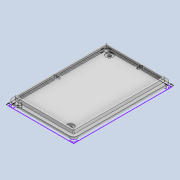
# Autodesk Inventor part: proper shit spodnji
Saved by Autodesk Inventor 2020 (Build 240168000, 168)
## iProperties
Created: 2020-08-03
Part Number: proper shit spodnji
Material: Generic
Document SubType Name: Modeling
Designer: borbu
Density: 1 g/cm^3
Appearance: Default
Author: borbu
Autodesk Inventor part; units mm, degrees
ref_plane "YZ Plane" through (0, 0, 0) normal (1, 0, 0) x (0, 1, 0)
ref_plane "XZ Plane" through (0, 0, 0) normal (0, 1, 0) x (-1, 0, 0)
ref_plane "XY Plane" through (0, 0, 0) normal (0, 0, 1) x (1, 0, 0)
sketch "Sketch1" plane through (0, 0, 0) normal (0, 1, 0) x (-1, 0, 0)
  line L0 (-25, 37.5) -> (25, 37.5)
  line L1 (25, 37.5) -> (25, -37.5)
  line L2 (25, -37.5) -> (-25, -37.5)
  line L3 (-25, -37.5) -> (-25, 37.5)
  line L4 (25, 37.5) -> (-25, -37.5) construction
  line L5 (-22.5, 35) -> (22.5, 35)
  line L6 (22.5, 35) -> (22.5, -35)
  line L7 (22.5, -35) -> (-22.5, -35)
  line L8 (-22.5, -35) -> (-22.5, 35)
  line L9 (22.5, 35) -> (-22.5, -35) construction
  line L10 (22.5, 35) -> (20, 35)
  line L11 (20, 35) -> (20, 32.5)
  line L12 (20, 32.5) -> (22.5, 32.5)
  line L13 (22.5, 32.5) -> (22.5, 35)
  arc A0 (22.5, 32.5) -> (20, 35) centre (20, 32.5) ccw
  line L14 (25, 37.5) -> (21.5, 37.5)
  line L15 (21.5, 37.5) -> (21.5, 34)
  line L16 (21.5, 34) -> (25, 34)
  line L17 (25, 34) -> (25, 37.5)
  line L18 (22.5, -35) -> (20, -35)
  line L19 (20, -35) -> (20, -32.5)
  line L20 (20, -32.5) -> (22.5, -32.5)
  line L21 (22.5, -32.5) -> (22.5, -35)
  line L22 (-22.5, -35) -> (-20, -35)
  line L23 (-20, -35) -> (-20, -32.5)
  line L24 (-20, -32.5) -> (-22.5, -32.5)
  line L25 (-22.5, -32.5) -> (-22.5, -35)
  line L26 (-22.5, 35) -> (-20, 35)
  line L27 (-20, 35) -> (-20, 32.5)
  line L28 (-20, 32.5) -> (-22.5, 32.5)
  line L29 (-22.5, 32.5) -> (-22.5, 35)
  arc A1 (-20, 35) -> (-22.5, 32.5) centre (-20, 32.5) ccw
  arc A2 (-22.5, -32.5) -> (-20, -35) centre (-20, -32.5) ccw
  arc A3 (20, -35) -> (22.5, -32.5) centre (20, -32.5) ccw
  arc A4 (25, 34) -> (21.5, 37.5) centre (21.5, 34) ccw
  line L30 (25, -37.5) -> (21.5, -37.5)
  line L31 (21.5, -37.5) -> (21.5, -34)
  line L32 (21.5, -34) -> (25, -34)
  line L33 (25, -34) -> (25, -37.5)
  line L34 (-25, -37.5) -> (-21.5, -37.5)
  line L35 (-21.5, -37.5) -> (-21.5, -34)
  line L36 (-21.5, -34) -> (-25, -34)
  line L37 (-25, -34) -> (-25, -37.5)
  line L38 (-25, 37.5) -> (-21.5, 37.5)
  line L39 (-21.5, 37.5) -> (-21.5, 34)
  line L40 (-21.5, 34) -> (-25, 34)
  line L41 (-25, 34) -> (-25, 37.5)
  arc A5 (-21.5, 37.5) -> (-25, 34) centre (-21.5, 34) ccw
  arc A6 (-25, -34) -> (-21.5, -37.5) centre (-21.5, -34) ccw
  arc A7 (21.5, -37.5) -> (25, -34) centre (21.5, -34) ccw
  point P0 (0, 0)
  point P1 (25, 34)
  point P2 (-25, -34)
  point P3 (-22.5, -32.5)
  point P4 (-22, -34)
  point P5 (-22.5, -34)
  point P6 (22.5, -32.5)
  dimension "d0" = 50
  dimension "d1" = 75
  dimension "d2" = 45
  dimension "d3" = 70
  dimension "d8" = 2.5
  dimension "d9" = 2.5
  constraints: 84 end point, 20 parallel, 16 point on circle, 10 horizontal, 10 perpendicular, 8 centre point, 8 coincident, 2 midpoint, 1 point on line
  measures "d0" distance of L1.end L2.end
  measures "d1" distance of L0.end L1.end
  measures "d2" distance of L6.end L7.end
  measures "d3" distance of L5.end L6.end
  measures "d8" distance of L12.end L11.end
  measures "d9" distance of L11.end L10.end
extrude "Extrusion3" add sketch "Sketch1" along normal blind 3.5 contours L0 L15 L5 L39 | L39 L5 L8 L40 A5 | L40 L8 L36 L3 | A4 L16 L6 L5 L15 | L39 A1 L40 L8 L5 | L5 A1 L39 | L36 L8 L7 L35 A6 | L40 A1 L8 | L15 A0 L5 | L5 L6 L16 A0 L15 | L1 L32 L6 L16 | L5 L11 L12 L6 L20 L19 L7 L23 L24 L8 L28 L27 | L27 L28 A1 L40 L39 | L39 L40 A1 | L36 A2 L35 L7 L8 | L8 A2 L36 | L35 L7 L31 L2 | A0 L15 L16 L12 L11 | A0 L16 L15 | A7 L31 L7 L6 L32 | L6 A0 L16 | L24 L23 A2 L35 L36 | L36 L35 A2 | L35 A2 L7 | L32 A3 L6 | L6 L7 L31 A3 L32 | L7 A3 L31 | A3 L32 L31 L19 L20 | A3 L31 L32
fillet "Fillet1" radius 3 8 edges at (-23.9749, 0, 36.4749) (0, 0, 37.5) (23.9749, 0, 36.4749) (25, 0, 0) (23.9749, 0, -36.4749) (0, 0, -37.5) (-23.9749, 0, -36.4749) (-25, 0, 0)
sketch "Sketch2" plane through (0, 3.5, 0) normal (0, 1, 0) x (1, 0, 0)
  arc A0 (20, 32.5) -> (17.5, 35) centre (17.5, 32.5) ccw projected
  line L0 (17.5, 35) -> (17.5, 33.5)
  line L1 (20, -32.5) -> (20, 32.5) projected
  line L2 (20, 32.5) -> (18.5, 32.5)
  line L3 (18.5, 32.5) -> (17.5, 33.5)
  line L4 (18, 33) -> (16.0555, 31.0555)
  circle A1 centre (16.0555, 31.0555) radius 2.75
  line L5 (-20, 32.5) -> (-20, -32.5) projected
  line L6 (-20, -32.5) -> (-18.5, -32.5)
  line L7 (-17.5, -35) -> (17.5, -35) projected
  line L8 (-17.5, -35) -> (-17.5, -33.5)
  line L9 (-17.5, -33.5) -> (-18.5, -32.5)
  line L10 (-18, -33) -> (-16.0555, -31.0555)
  line L11 (-18, -33) -> (-15.25, -33) construction
  circle A2 centre (-16.0555, -31.0555) radius 2.75
  arc A3 (17.5812, 28.7675) -> (18.8055, 31.0555) centre (16.0555, 31.0555) ccw construction
  arc A4 (17.8504, 28.3639) -> (19.2906, 31.0555) centre (16.0555, 31.0555) ccw
  arc A5 (17.3121, 29.1712) -> (18.3203, 31.0555) centre (16.0555, 31.0555) ccw
  arc A6 (17.3121, 29.1712) -> (17.8504, 28.3639) centre (17.5812, 28.7675) ccw
  arc A7 (19.2906, 31.0555) -> (18.3203, 31.0555) centre (18.8055, 31.0555) ccw
  arc A8 (14.2605, 33.747) -> (12.8203, 31.0555) centre (16.0555, 31.0555) ccw
  arc A9 (12.8203, 31.0555) -> (13.7906, 31.0555) centre (13.3055, 31.0555) ccw
  arc A10 (14.7989, 32.9398) -> (14.2605, 33.747) centre (14.5297, 33.3434) ccw
  arc A11 (14.7989, 32.9398) -> (13.7906, 31.0555) centre (16.0555, 31.0555) ccw
  arc A12 (-14.2605, -33.747) -> (-12.8203, -31.0555) centre (-16.0555, -31.0555) ccw
  arc A13 (-14.7989, -32.9398) -> (-13.7906, -31.0555) centre (-16.0555, -31.0555) ccw
  arc A14 (-14.7989, -32.9398) -> (-14.2605, -33.747) centre (-14.5297, -33.3434) ccw
  arc A15 (-12.8203, -31.0555) -> (-13.7906, -31.0555) centre (-13.3055, -31.0555) ccw
  arc A16 (-17.8504, -28.3639) -> (-19.2906, -31.0555) centre (-16.0555, -31.0555) ccw
  arc A17 (-19.2906, -31.0555) -> (-18.3203, -31.0555) centre (-18.8055, -31.0555) ccw
  arc A18 (-17.3121, -29.1712) -> (-17.8504, -28.3639) centre (-17.5812, -28.7675) ccw
  arc A19 (-17.3121, -29.1712) -> (-18.3203, -31.0555) centre (-16.0555, -31.0555) ccw
  line L12 (-19.2843, -34.2843) -> (-16.7157, -31.7157) construction
  line L13 (-18.86, -34.7085) -> (-16.2915, -32.14)
  line L14 (-17.14, -31.2915) -> (-19.7085, -33.86)
  arc A20 (-19.7085, -33.86) -> (-18.86, -34.7085) centre (-19.2843, -34.2843) ccw
  arc A21 (-16.2915, -32.14) -> (-17.14, -31.2915) centre (-16.7157, -31.7157) ccw
  line L15 (16.5205, 31.5205) -> (19.4795, 34.4795) construction
  line L16 (16.9448, 31.0962) -> (19.9038, 34.0552)
  line L17 (19.0552, 34.9038) -> (16.0962, 31.9448)
  arc A22 (16.0962, 31.9448) -> (16.9448, 31.0962) centre (16.5205, 31.5205) ccw
  arc A23 (19.9038, 34.0552) -> (19.0552, 34.9038) centre (19.4795, 34.4795) ccw
  circle A24 centre (16.0555, 31.0555) radius 1.25
  circle A25 centre (-16.0555, -31.0555) radius 1.25
  line L18 (21.5, 34.5) -> (-21.5, 34.5) projected
  line L19 (0, 34.5) -> (0, -35)
  circle A26 centre (16.0555, -31.0555) radius 2.75
  circle A27 centre (16.0555, -31.0555) radius 1.25
  circle A28 centre (-16.0555, 31.0555) radius 2.75
  circle A29 centre (-16.0555, 31.0555) radius 1.25
  point P0 (0, 0)
  point P1 (18.3774, 32.5289)
  point P2 (17.5289, 33.3774)
  point P3 (14.9555, 33.5759)
  point P4 (13.3482, 30.5722)
  point P5 (17.1554, 28.535)
  point P6 (18.7627, 31.5387)
  point P7 (-18.3774, -32.5289)
  point P8 (-17.5289, -33.3774)
  point P9 (-14.9555, -33.5759)
  point P10 (-13.3482, -30.5722)
  point P11 (-17.1554, -28.535)
  point P12 (-18.7627, -31.5387)
  dimension "d32" = 5.5
  dimension "d29" = 1.5
  dimension "d30" = 1.5
  dimension "d31" = 2.75
  dimension "d33" = 1.5
  dimension "d34" = 1.5
  dimension "d35" = 2.75
  dimension "d36" = 45
  dimension "d37" = 5.5
  dimension "d40" = 360
  dimension "d44" = 1.2
  dimension "d45" = 1.2
  dimension "d60" = 2.5
  dimension "d61" = 2.5
  constraints: 42 point on circle, 36 end point, 28 centre point, 16 tangent, 6 midpoint, 5 coincident, 4 symmetric about line, 3 horizontal, 3 point on line, 2 parallel, 2 perpendicular, 2 vertical, 1 equal length, 32 other
  measures "d29" distance of L0.start L0.end
  measures "d30" distance of L1.end L2.end
  measures "d31" distance of L4.start L4.end
  measures "d33" distance of L5.end L6.end
  measures "d34" distance of L7.start L8.end
  measures "d35" distance of L10.start L10.end
  measures "d36" angle of L11 L10
  measures "d37" diameter of A2
  measures "d44" diameter of A21
  measures "d45" diameter of A23
  measures "d60" diameter of A24
  measures "d61" diameter of A25
sketch "Sketch4" plane through (0, 3.5, 0) normal (0, 1, 0) x (1, 0, 0)
  line L0 (-22, 34.5263) -> (22, 34.5263)
  line L1 (22, 34.5263) -> (22, -34.5263)
  line L2 (22, -34.5263) -> (-22, -34.5263)
  line L3 (-22, -34.5263) -> (-22, 34.5263)
  line L4 (-22, 34.5263) -> (22, -34.5263) construction
  line L5 (22, 34.5263) -> (-22, -34.5263) construction
  line L6 (21.5, 34.5) -> (-21.5, 34.5) projected
  line L7 (-21.5, 34.5) -> (-21.5, 37.5) projected
  line L8 (17.5001, 34.5) -> (-21.5, 34.5) construction
  line L9 (22, -34) -> (22, 34) projected
  line L10 (22, 32.5003) -> (22, -34.5263) construction
  arc A0 (21.5, -34.5263) -> (22.5, -34.5263) centre (22, -34.5263) ccw
  line L11 (22, -34.5263) -> (-22, -34.5263) construction
  line L12 (22, -34.0263) -> (-22, -34.0263)
  line L13 (-22, -35.0263) -> (22, -35.0263)
  arc A1 (22, -35.0263) -> (22, -34.0263) centre (22, -34.5263) ccw
  arc A2 (-22, -34.0263) -> (-22, -35.0263) centre (-22, -34.5263) ccw
  line L14 (-22, -34.5263) -> (-22, 34.5263) construction
  line L15 (-21.5, -34.5263) -> (-21.5, 34.5263)
  line L16 (-22.5, 34.5263) -> (-22.5, -34.5263)
  arc A3 (-22.5, -34.5263) -> (-21.5, -34.5263) centre (-22, -34.5263) ccw
  arc A4 (-21.5, 34.5263) -> (-22.5, 34.5263) centre (-22, 34.5263) ccw
  line L17 (22, 34.5263) -> (-22, 34.5263) construction
  line L18 (22, 35.0263) -> (-22, 35.0263)
  line L19 (-22, 34.0263) -> (22, 34.0263)
  arc A5 (22, 34.0263) -> (22, 35.0263) centre (22, 34.5263) ccw
  arc A6 (-22, 35.0263) -> (-22, 34.0263) centre (-22, 34.5263) ccw
  line L20 (22, -34.5263) -> (22, 34.5263) construction
  line L21 (22.5, -34.5263) -> (22.5, 34.5263)
  line L22 (21.5, 34.5263) -> (21.5, -34.5263)
  arc A7 (21.5, -34.5263) -> (22.5, -34.5263) centre (22, -34.5263) ccw
  arc A8 (22.5, 34.5263) -> (21.5, 34.5263) centre (22, 34.5263) ccw
  point P0 (0, 0)
  point P1 (-1.9999, 34.5)
  point P2 (22, -1.013)
  point P3 (0, -34.5263)
  point P4 (-22, 0)
  point P5 (0, 34.5263)
  point P6 (22, 0)
  point P7 (-22.5, -34.5263)
  point P8 (22, -35.0263)
  point P9 (22.5, -34.5263)
  point P10 (22.5, 34.5263)
  point P11 (-21.5, -34.0263)
  point P12 (-21.5, 34.0263)
  point P13 (21.5, 34.0263)
  point P14 (21.5, -34.0263)
  dimension "d68" = 1
  dimension "d69" = 1
  dimension "d70" = 1
  dimension "d71" = 1
  dimension "d72" = 1
  constraints: 50 end point, 18 point on circle, 16 tangent, 9 centre point, 8 midpoint, 6 parallel, 2 collinear, 2 perpendicular, 2 point on line, 1 horizontal, 1 vertical, 3 other
  measures "d68" diameter of A0
  measures "d69" diameter of A2
  measures "d70" diameter of A4
  measures "d71" diameter of A6
  measures "d72" diameter of A8
extrude "Extrusion11" add sketch "Sketch4" along normal blind 3 contours L3 A6 A4 L0 | L0 L7 L15 L19 L3 | L7 L18 A8 L0 | L0 L22 L6 L7 | A4 L18 L7 | L19 L15 L12 L3 | L3 A2 L16 A6 | A8 A5 L1 L0 | L0 L1 L19 L22 | L6 L22 L19 L15 | L12 L15 L2 L3 | L3 L2 A3 A2 | L12 L22 L2 L15 | L19 L1 L12 L22 | A5 L21 A1 L1 | L2 A0 L13 A3 | L12 L1 L2 L22 | A0 L2 L1 A1
fillet "Fillet2" radius 0.5 12 edges at (-22.3536, 6.5, -34.8799) (-22.5, 6.5, 0) (-22.3536, 6.5, 34.8799) (0, 6.5, 35.0263) (22.3536, 6.5, 34.8799) (22.5, 6.5, 0) (22.3536, 6.5, -34.8799) (0, 6.5, -35.0263) (0, 6.5, -34.0263) (21.5, 6.5, 0) (0, 6.5, 34.0263) (-21.5, 6.5, 0)
extrude "Extrusion12" cut sketch "Sketch2" against normal blind 0.5 contours A26 | A28
sketch "Sketch6" plane through (0, 3.5, 0) normal (0, 1, 0) x (1, 0, 0)
  circle A0 centre (16.0555, -31.0555) radius 1.25 projected
  circle A1 centre (16.0555, -31.0555) radius 1.25
  point P0 (0, 0)
  constraints: 1 centre point, 1 coincident
extrude "Extrusion13" cut sketch "Sketch6" against normal blind 5
sketch "Sketch7" plane through (-16.0555, 3.5, -31.0555) normal (0, 1, 0) x (1, 0, 0)
  circle A0 centre (0, 0) radius 1.25
  point P0 (16.0555, -31.0555)
  constraints: 1 centre point
extrude "Extrusion14" cut sketch "Sketch7" against normal blind 5
chamfer "Chamfer2" distance 0.5 angle 45 2 edges at (14.8055, 0, 31.0555) (-17.3055, 0, -31.0555)
body "Solid2"
